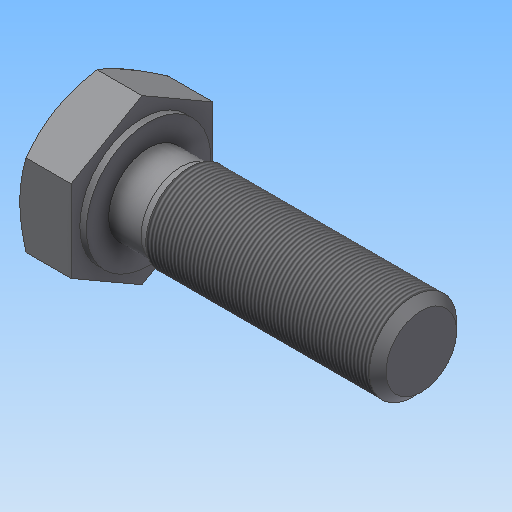
# Autodesk Inventor part: DIN 933 - M8  x 25
Saved by Autodesk Inventor 2020.1 (Build 241239000, 239)
## iProperties
Comments: To add or edit properties for Autodesk Inventor files, use iProperties.
Shininess: 64.0
Length Units: 11269
Angle Units: 11279
Time Units: 11290
Mass Units: 11283
Length Display Precision: 3
Angle Display Precision: 2
Compacted: True
Alert: To add or edit properties for Autodesk Inventor files, use iProperties.
Library Location: C:\ap\Inventor 6\content
Library: local
SubLibrary: DIN
Family: 19
Member: 166
Member Major Revision: 1
Member Minor Revision: 1
Created: 2003-02-27
Part Number: DIN 933 - M8  x 25
Vendor: Autodesk Inc.
Document SubType Name: Modeling
Designer: Joe M
Description: Sechskantschraube
Standard: DIN 933 M8  x 25
Engineer: Joe M
Material: Generic
Density: 1 g/cm^3
Appearance: Default
Density: 0.0
Volumn: 0.0
Area: 0.0
PropertySet Name: Model Information
Control State: 0
Master: False
Checked Out: False
Author: Joe M
Autodesk Inventor part; units mm, degrees
ref_plane "YZ Plane" through (0, 0, 0) normal (1, 0, 0) x (0, 1, 0)
ref_plane "XZ Plane" through (0, 0, 0) normal (0, 1, 0) x (-1, 0, 0)
ref_plane "XY Plane" through (0, 0, 0) normal (0, 0, 1) x (1, 0, 0)
sketch "Skizze1" plane through (0, 0, 0) normal (0, 0, 1) x (1, 0, 0)
  line L0 (0, 5.7) -> (0, 3.6617)
  line L1 (3.75, 4) -> (25, 4)
  line L2 (25, 4) -> (25, 0)
  line L3 (25, 0) -> (-0.6001, 0)
  line L4 (-0.4751, 0) -> (2.675, 0) projected
  line L5 (-0.6001, 0) -> (-0.6001, 5.7)
  line L6 (-0.6001, 5.7) -> (0, 5.7)
  line L7 (3.75, 4) -> (2.9831, 3.6617)
  line L8 (2.9831, 3.6617) -> (0, 3.6617)
  line L9 (0, -0.1135) -> (0, 1.4755) projected
  dimension "d0" = 25
  dimension "d1" = 21.25
  dimension "d2" = 8
  dimension "d9" = 0.6001
  dimension "d10" = 11.4
  dimension "d13" = 0.7669
  dimension "d14" = 7.3234
  constraints: 16 end point, 2 collinear, 2 perpendicular, 1 parallel
  measures "d0" distance between parallel lines of L2 L0
  measures "d1" distance from line of L1.start L2
  measures "d2" diameter of L1 L3
  measures "d9" distance between parallel lines of L5 L0
  measures "d10" diameter of L6 L3
  measures "d13" horizontal distance of L1.start L7.end
  measures "d14" diameter of L8 L3
revolve "Körper" add sketch "Skizze1" angle 360 about axis through (25, 0, 0) along (-1, 0, 0)
sketch "Skizze2" plane through (-0.6001, 0, 0) normal (-1, 0, 0) x (0, 0, 1)
  line L0 (0, 7.5056) -> (6.5, 3.7528)
  line L1 (6.5, 3.7528) -> (6.5, -3.7528)
  line L2 (6.5, -3.7528) -> (0, -7.5056)
  line L3 (0, -7.5056) -> (-6.5, -3.7528)
  line L4 (-6.5, -3.7528) -> (-6.5, 3.7528)
  line L5 (-6.5, 3.7528) -> (0, 7.5056)
  point P0 (0, 0)
  point P1 (0, 0)
  dimension "d11" = 13
  constraints: 12 end point, 1 coincident, 1 vertical, 11 other
  measures "d11" distance between parallel lines of L4 L1
extrude "Kopf" add sketch "Skizze2" along normal blind 4.7
sketch "Skizze4" plane through (0, 0, 0) normal (0, 0, 1) x (1, 0, 0)
  line L0 (-5.3001, 6.5) -> (-5.3001, 7.5056)
  line L1 (-5.3001, 7.5056) -> (-4.7195, 7.5056)
  line L2 (-4.7195, 7.5056) -> (-5.3001, 6.5)
  line L3 (-1.1851, 0) -> (0.0049, 0) projected
  line L4 (-0.6001, 7.5056) -> (-5.3001, 7.5056) projected
  line L5 (-5.3001, 3.7528) -> (-5.3001, 7.5056) projected
  dimension "d5" = 30
  dimension "d19" = 13
  constraints: 6 end point, 2 collinear, 1 perpendicular, 1 vertical
  measures "d5" angle of L2 L0
  measures "d19" diameter of L0.start L3
revolve "Fase1" cut sketch "Skizze4" angle 360 about axis through (-10, 0, 0) along (1, 0, 0)
thread "Gewinde" size "M1.6x0.35" class "6g" standard "ANSI Metric M Profile" length 21.25
chamfer "Fase2" distance 0.7668 distance2 0.7669 1 edges at (25, -4, 0) measured on face at (25, 0.998, -0.8842)
equation "\"d0\" = NLG"
equation "\"d1\" = GEL"
equation "\"d2\" = GD"
equation "\"d10\" = SD2"
equation "\"d14\" = BDM"
equation "\"d11\" = SW"
equation "\"d3\" = KOH - SD"
equation "\"d5\" = ANG1"
equation "\"d19\" = SW0"
equation "\"d15\" = GEL"
equation "\"d6\" = -0.5 * SPD + 0.5 * GD"
equation "\"NLG\" = 25"
equation "\"GD\" = NND"
equation "\"BDM\" = 7.32342"
equation "\"KOH\" = 5.3"
equation "\"GEL\" = 21.25"
equation "\"SW\" = 13"
equation "\"SW0\" = 13"
equation "\"SPD\" = NND - 1.2269 * TPU"
equation "\"SD2\" = 11.4"
equation "\"SD\" = 0.6"
equation "\"ANG1\" = 30deg"
equation "\"GAL\" = 0.61345 * TPU"
equation "\"GUL\" = 0.61345 * TPU"
equation "\"RR\" = 0.4"
equation "\"d20\" = -NLG"
equation "\"TOA\" = 30deg"
equation "\"PTC\" = TPU"
equation "\"GD1\" = THREADDIA - 1.2269 * TPU"
equation "\"TPU\" = 1.25"
equation "\"THREADDIA\" = 8"
equation "\"E0\" = 1.155 * SW"
equation "\"NND\" = 8"
body "Solid1"
